Autodesk Inventor part; units mm, degrees
(part 3 of 3)
sketch "Sketch3" plane through (0, 0, 0) normal (-1, 0, 0) x (0, 0, 1)
  line L0 (70.1139, 246.1211) -> (70.1139, 280.6833) projected
  line L1 (70.1139, 280.6833) -> (54.8144, 280.6833) projected
  line L2 (54.8144, 280.6833) -> (54.8144, 296.1211) projected
  line L3 (54.8144, 296.1211) -> (81.2199, 296.1211) projected
  line L4 (81.2199, 296.1211) -> (87.7637, 289.6234) projected
  line L5 (87.7637, 289.6234) -> (87.7637, 252.6188) projected
  line L6 (87.7637, 252.6188) -> (81.266, 246.1211) projected
  line L7 (81.266, 246.1211) -> (70.1139, 246.1211) projected
  line L8 (109.8374, 246.075) -> (109.8374, 261.8815) projected
  line L9 (109.8374, 261.8815) -> (125.1369, 261.8815) projected
  line L10 (125.1369, 261.8815) -> (125.1369, 296.1211) projected
  line L11 (125.1369, 296.1211) -> (142.7867, 296.1211) projected
  line L12 (142.7867, 296.1211) -> (142.7867, 262.6649) projected
  line L13 (142.7867, 262.6649) -> (126.1968, 246.075) projected
  line L14 (126.1968, 246.075) -> (109.8374, 246.075) projected
  line L15 (145.5517, 246.1211) -> (145.5517, 260.9137) projected
  line L16 (145.5517, 260.9137) -> (178.501, 260.9137) projected
  line L17 (178.501, 260.9137) -> (178.501, 246.1211) projected
  line L18 (178.501, 246.1211) -> (145.5517, 246.1211) projected
  line L19 (180.5286, 246.1211) -> (180.5286, 296.1211) projected
  line L20 (180.5286, 296.1211) -> (191.5885, 296.1211) projected
  line L21 (191.5885, 296.1211) -> (198.0862, 289.6234) projected
  line L22 (198.0862, 289.6234) -> (198.0862, 252.6188) projected
  line L23 (198.0862, 252.6188) -> (191.5885, 246.1211) projected
  line L24 (191.5885, 246.1211) -> (180.5286, 246.1211) projected
  line L25 (220.4365, 246.1672) -> (220.4365, 260.9598) projected
  line L26 (220.4365, 260.9598) -> (235.736, 260.9598) projected
  line L27 (235.736, 260.9598) -> (235.736, 282.204) projected
  line L28 (235.736, 282.204) -> (253.3858, 282.204) projected
  line L29 (253.3858, 282.204) -> (253.3858, 254.2317) projected
  line L30 (253.3858, 254.2317) -> (245.3213, 246.1672) projected
  line L31 (245.3213, 246.1672) -> (220.4365, 246.1672) projected
  line L32 (301.9111, 246.1211) -> (290.9895, 246.1211) projected
  line L33 (290.9895, 246.1211) -> (290.9895, 296.1211) projected
  line L34 (290.9895, 296.1211) -> (308.4088, 296.1211) projected
  line L35 (308.4088, 296.1211) -> (308.4088, 252.6188) projected
  line L36 (308.4088, 252.6188) -> (301.9111, 246.1211) projected
  line L37 (288.9618, 246.1211) -> (256.1508, 246.1211) projected
  line L38 (256.1508, 246.1211) -> (256.1508, 260.9137) projected
  line L39 (256.1508, 260.9137) -> (288.9618, 260.9137) projected
  line L40 (288.9618, 260.9137) -> (288.9618, 246.1211) projected
  line L41 (200.8512, 246.1672) -> (200.8512, 282.204) projected
  line L42 (200.8512, 282.204) -> (218.501, 282.204) projected
  line L43 (218.501, 282.204) -> (218.501, 246.1672) projected
  line L44 (218.501, 246.1672) -> (200.8512, 246.1672) projected
  line L45 (145.5517, 280.6833) -> (145.5517, 296.1211) projected
  line L46 (145.5517, 296.1211) -> (178.501, 296.1211) projected
  line L47 (178.501, 296.1211) -> (178.501, 280.6833) projected
  line L48 (178.501, 280.6833) -> (145.5517, 280.6833) projected
  line L49 (145.5517, 266.5358) -> (145.5517, 278.6557) projected
  line L50 (145.5517, 278.6557) -> (178.501, 278.6557) projected
  line L51 (178.501, 278.6557) -> (178.501, 266.5358) projected
  line L52 (178.501, 266.5358) -> (145.5517, 266.5358) projected
  line L53 (107.9019, 246.1211) -> (90.5286, 262.757) projected
  line L54 (90.5286, 262.757) -> (90.5286, 296.1211) projected
  line L55 (90.5286, 296.1211) -> (107.9019, 296.1211) projected
  line L56 (107.9019, 296.1211) -> (107.9019, 246.1211) projected
  line L57 (35.2291, 252.6649) -> (35.2291, 289.5773) projected
  line L58 (35.2291, 289.5773) -> (41.7729, 296.1211) projected
  line L59 (41.7729, 296.1211) -> (52.8789, 296.1211) projected
  line L60 (52.8789, 296.1211) -> (52.8789, 260.9137) projected
  line L61 (52.8789, 260.9137) -> (68.2706, 260.9137) projected
  line L62 (68.2706, 260.9137) -> (68.2706, 246.1211) projected
  line L63 (68.2706, 246.1211) -> (41.7729, 246.1211) projected
  line L64 (41.7729, 246.1211) -> (35.2291, 252.6649) projected
  line L65 (-22.4898, 96.0981) -> (-22.4898, 576.0981) projected
  line L66 (367.5102, 96.0981) -> (-22.4898, 96.0981) projected
  line L67 (367.5102, 576.0981) -> (367.5102, 96.0981) projected
  line L68 (-22.4898, 576.0981) -> (367.5102, 576.0981) projected
  circle A0 centre (42.5102, 103.5981) radius 1.75 projected
  circle A1 centre (302.5102, 568.5981) radius 1.75 projected
  circle A2 centre (42.5102, 568.5981) radius 1.75 projected
  circle A3 centre (360.0102, 161.0981) radius 1.75 projected
  circle A4 centre (360.0102, 511.0981) radius 1.75 projected
  circle A5 centre (-14.9898, 161.0981) radius 1.75 projected
  circle A6 centre (-14.9898, 511.0981) radius 1.75 projected
  circle A7 centre (172.5102, 568.5981) radius 1.75 projected
  circle A8 centre (302.5102, 103.5981) radius 1.75 projected
  line L69 (-2.265, 163.0981) -> (3.5085, 163.0981) projected
  line L70 (-5.1518, 168.0981) -> (-2.265, 163.0981) projected
  line L71 (-2.265, 173.0981) -> (-5.1518, 168.0981) projected
  line L72 (3.5085, 173.0981) -> (-2.265, 173.0981) projected
  line L73 (6.3952, 168.0981) -> (3.5085, 173.0981) projected
  line L74 (3.5085, 163.0981) -> (6.3952, 168.0981) projected
  line L75 (23.735, 143.0981) -> (20.8482, 138.0981) projected
  line L76 (29.5085, 143.0981) -> (23.735, 143.0981) projected
  line L77 (32.3952, 138.0981) -> (29.5085, 143.0981) projected
  line L78 (29.5085, 133.0981) -> (32.3952, 138.0981) projected
  line L79 (23.735, 133.0981) -> (29.5085, 133.0981) projected
  line L80 (20.8482, 138.0981) -> (23.735, 133.0981) projected
  line L81 (45.3856, 160.5981) -> (42.4988, 165.5981) projected
  line L82 (42.4988, 155.5981) -> (45.3856, 160.5981) projected
  line L83 (36.7253, 155.5981) -> (42.4988, 155.5981) projected
  line L84 (33.8386, 160.5981) -> (36.7253, 155.5981) projected
  line L85 (36.7253, 165.5981) -> (33.8386, 160.5981) projected
  line L86 (42.4988, 165.5981) -> (36.7253, 165.5981) projected
  line L87 (55.5085, 128.0981) -> (49.735, 128.0981) projected
  line L88 (58.3952, 123.0981) -> (55.5085, 128.0981) projected
  line L89 (55.5085, 118.0981) -> (58.3952, 123.0981) projected
  line L90 (49.735, 118.0981) -> (55.5085, 118.0981) projected
  line L91 (46.8482, 123.0981) -> (49.735, 118.0981) projected
  line L92 (49.735, 128.0981) -> (46.8482, 123.0981) projected
  line L93 (72.8482, 168.0981) -> (75.735, 163.0981) projected
  line L94 (75.735, 173.0981) -> (72.8482, 168.0981) projected
  line L95 (81.5085, 173.0981) -> (75.735, 173.0981) projected
  line L96 (84.3952, 168.0981) -> (81.5085, 173.0981) projected
  line L97 (81.5085, 163.0981) -> (84.3952, 168.0981) projected
  line L98 (75.735, 163.0981) -> (81.5085, 163.0981) projected
  line L99 (97.3856, 130.5981) -> (94.4988, 135.5981) projected
  line L100 (94.4988, 125.5981) -> (97.3856, 130.5981) projected
  line L101 (88.7253, 125.5981) -> (94.4988, 125.5981) projected
  line L102 (85.8386, 130.5981) -> (88.7253, 125.5981) projected
  line L103 (88.7253, 135.5981) -> (85.8386, 130.5981) projected
  line L104 (94.4988, 135.5981) -> (88.7253, 135.5981) projected
  line L105 (107.5085, 158.0981) -> (101.735, 158.0981) projected
  line L106 (110.3952, 153.0981) -> (107.5085, 158.0981) projected
  line L107 (107.5085, 148.0981) -> (110.3952, 153.0981) projected
  line L108 (101.735, 148.0981) -> (107.5085, 148.0981) projected
  line L109 (98.8482, 153.0981) -> (101.735, 148.0981) projected
  line L110 (101.735, 158.0981) -> (98.8482, 153.0981) projected
  line L111 (120.4988, 140.5981) -> (123.3856, 145.5981) projected
  line L112 (114.7253, 140.5981) -> (120.4988, 140.5981) projected
  line L113 (111.8386, 145.5981) -> (114.7253, 140.5981) projected
  line L114 (114.7253, 150.5981) -> (111.8386, 145.5981) projected
  line L115 (120.4988, 150.5981) -> (114.7253, 150.5981) projected
  line L116 (123.3856, 145.5981) -> (120.4988, 150.5981) projected
  line L117 (127.735, 143.0981) -> (124.8482, 138.0981) projected
  line L118 (133.5085, 143.0981) -> (127.735, 143.0981) projected
  line L119 (136.3952, 138.0981) -> (133.5085, 143.0981) projected
  line L120 (133.5085, 133.0981) -> (136.3952, 138.0981) projected
  line L121 (127.735, 133.0981) -> (133.5085, 133.0981) projected
  line L122 (124.8482, 138.0981) -> (127.735, 133.0981) projected
  line L123 (153.735, 143.0981) -> (150.8482, 138.0981) projected
  line L124 (159.5085, 143.0981) -> (153.735, 143.0981) projected
  line L125 (162.3952, 138.0981) -> (159.5085, 143.0981) projected
  line L126 (159.5085, 133.0981) -> (162.3952, 138.0981) projected
  line L127 (153.735, 133.0981) -> (159.5085, 133.0981) projected
  line L128 (150.8482, 138.0981) -> (153.735, 133.0981) projected
  line L129 (159.5085, 158.0981) -> (153.735, 158.0981) projected
  line L130 (162.3952, 153.0981) -> (159.5085, 158.0981) projected
  line L131 (159.5085, 148.0981) -> (162.3952, 153.0981) projected
  line L132 (153.735, 148.0981) -> (159.5085, 148.0981) projected
  line L133 (150.8482, 153.0981) -> (153.735, 148.0981) projected
  line L134 (153.735, 158.0981) -> (150.8482, 153.0981) projected
  line L135 (176.8482, 168.0981) -> (179.735, 163.0981) projected
  line L136 (179.735, 173.0981) -> (176.8482, 168.0981) projected
  line L137 (185.5085, 173.0981) -> (179.735, 173.0981) projected
  line L138 (188.3952, 168.0981) -> (185.5085, 173.0981) projected
  line L139 (185.5085, 163.0981) -> (188.3952, 168.0981) projected
  line L140 (179.735, 163.0981) -> (185.5085, 163.0981) projected
  line L141 (201.3856, 130.5981) -> (198.4988, 135.5981) projected
  line L142 (198.4988, 125.5981) -> (201.3856, 130.5981) projected
  line L143 (192.7253, 125.5981) -> (198.4988, 125.5981) projected
  line L144 (189.8386, 130.5981) -> (192.7253, 125.5981) projected
  line L145 (192.7253, 135.5981) -> (189.8386, 130.5981) projected
  line L146 (198.4988, 135.5981) -> (192.7253, 135.5981) projected
  line L147 (211.5085, 158.0981) -> (205.735, 158.0981) projected
  line L148 (214.3952, 153.0981) -> (211.5085, 158.0981) projected
  line L149 (211.5085, 148.0981) -> (214.3952, 153.0981) projected
  line L150 (205.735, 148.0981) -> (211.5085, 148.0981) projected
  line L151 (202.8482, 153.0981) -> (205.735, 148.0981) projected
  line L152 (205.735, 158.0981) -> (202.8482, 153.0981) projected
  line L153 (224.4988, 140.5981) -> (227.3856, 145.5981) projected
  line L154 (218.7253, 140.5981) -> (224.4988, 140.5981) projected
  line L155 (215.8386, 145.5981) -> (218.7253, 140.5981) projected
  line L156 (218.7253, 150.5981) -> (215.8386, 145.5981) projected
  line L157 (224.4988, 150.5981) -> (218.7253, 150.5981) projected
  line L158 (227.3856, 145.5981) -> (224.4988, 150.5981) projected
  line L159 (231.735, 143.0981) -> (228.8482, 138.0981) projected
  line L160 (237.5085, 143.0981) -> (231.735, 143.0981) projected
  line L161 (240.3952, 138.0981) -> (237.5085, 143.0981) projected
  line L162 (237.5085, 133.0981) -> (240.3952, 138.0981) projected
  line L163 (231.735, 133.0981) -> (237.5085, 133.0981) projected
  line L164 (228.8482, 138.0981) -> (231.735, 133.0981) projected
  line L165 (253.3856, 160.5981) -> (250.4988, 165.5981) projected
  line L166 (250.4988, 155.5981) -> (253.3856, 160.5981) projected
  line L167 (244.7253, 155.5981) -> (250.4988, 155.5981) projected
  line L168 (241.8386, 160.5981) -> (244.7253, 155.5981) projected
  line L169 (244.7253, 165.5981) -> (241.8386, 160.5981) projected
  line L170 (250.4988, 165.5981) -> (244.7253, 165.5981) projected
  line L171 (263.5085, 128.0981) -> (257.735, 128.0981) projected
  line L172 (266.3952, 123.0981) -> (263.5085, 128.0981) projected
  line L173 (263.5085, 118.0981) -> (266.3952, 123.0981) projected
  line L174 (257.735, 118.0981) -> (263.5085, 118.0981) projected
  line L175 (254.8482, 123.0981) -> (257.735, 118.0981) projected
  line L176 (257.735, 128.0981) -> (254.8482, 123.0981) projected
  line L177 (315.5085, 128.0981) -> (309.735, 128.0981) projected
  line L178 (318.3952, 123.0981) -> (315.5085, 128.0981) projected
  line L179 (315.5085, 118.0981) -> (318.3952, 123.0981) projected
  line L180 (309.735, 118.0981) -> (315.5085, 118.0981) projected
  line L181 (306.8482, 123.0981) -> (309.735, 118.0981) projected
  line L182 (309.735, 128.0981) -> (306.8482, 123.0981) projected
  line L183 (341.5085, 158.0981) -> (335.735, 158.0981) projected
  line L184 (344.3952, 153.0981) -> (341.5085, 158.0981) projected
  line L185 (341.5085, 148.0981) -> (344.3952, 153.0981) projected
  line L186 (335.735, 148.0981) -> (341.5085, 148.0981) projected
  line L187 (332.8482, 153.0981) -> (335.735, 148.0981) projected
  line L188 (335.735, 158.0981) -> (332.8482, 153.0981) projected
  line L189 (280.8482, 168.0981) -> (283.735, 163.0981) projected
  line L190 (283.735, 173.0981) -> (280.8482, 168.0981) projected
  line L191 (289.5085, 173.0981) -> (283.735, 173.0981) projected
  line L192 (292.3952, 168.0981) -> (289.5085, 173.0981) projected
  line L193 (289.5085, 163.0981) -> (292.3952, 168.0981) projected
  line L194 (283.735, 163.0981) -> (289.5085, 163.0981) projected
  line L195 (283.735, 143.0981) -> (280.8482, 138.0981) projected
  line L196 (289.5085, 143.0981) -> (283.735, 143.0981) projected
  line L197 (292.3952, 138.0981) -> (289.5085, 143.0981) projected
  line L198 (289.5085, 133.0981) -> (292.3952, 138.0981) projected
  line L199 (283.735, 133.0981) -> (289.5085, 133.0981) projected
  line L200 (280.8482, 138.0981) -> (283.735, 133.0981) projected
  line L201 (309.735, 143.0981) -> (306.8482, 138.0981) projected
  line L202 (315.5085, 143.0981) -> (309.735, 143.0981) projected
  line L203 (318.3952, 138.0981) -> (315.5085, 143.0981) projected
  line L204 (315.5085, 133.0981) -> (318.3952, 138.0981) projected
  line L205 (309.735, 133.0981) -> (315.5085, 133.0981) projected
  line L206 (306.8482, 138.0981) -> (309.735, 133.0981) projected
  line L207 (3.5085, 128.0981) -> (-2.265, 128.0981) projected
  line L208 (6.3952, 123.0981) -> (3.5085, 128.0981) projected
  line L209 (3.5085, 118.0981) -> (6.3952, 123.0981) projected
  line L210 (-2.265, 118.0981) -> (3.5085, 118.0981) projected
  line L211 (-5.1518, 123.0981) -> (-2.265, 118.0981) projected
  line L212 (-2.265, 128.0981) -> (-5.1518, 123.0981) projected
  line L213 (10.7253, 140.5981) -> (16.4988, 140.5981) projected
  line L214 (7.8386, 145.5981) -> (10.7253, 140.5981) projected
  line L215 (10.7253, 150.5981) -> (7.8386, 145.5981) projected
  line L216 (16.4988, 150.5981) -> (10.7253, 150.5981) projected
  line L217 (19.3856, 145.5981) -> (16.4988, 150.5981) projected
  line L218 (16.4988, 140.5981) -> (19.3856, 145.5981) projected
  line L219 (328.4988, 140.5981) -> (331.3856, 145.5981) projected
  line L220 (322.7253, 140.5981) -> (328.4988, 140.5981) projected
  line L221 (319.8386, 145.5981) -> (322.7253, 140.5981) projected
  line L222 (322.7253, 150.5981) -> (319.8386, 145.5981) projected
  line L223 (328.4988, 150.5981) -> (322.7253, 150.5981) projected
  line L224 (331.3856, 145.5981) -> (328.4988, 150.5981) projected
  line L225 (302.4988, 140.5981) -> (305.3856, 145.5981) projected
  line L226 (296.7253, 140.5981) -> (302.4988, 140.5981) projected
  line L227 (293.8386, 145.5981) -> (296.7253, 140.5981) projected
  line L228 (296.7253, 150.5981) -> (293.8386, 145.5981) projected
  line L229 (302.4988, 150.5981) -> (296.7253, 150.5981) projected
  line L230 (305.3856, 145.5981) -> (302.4988, 150.5981) projected
  line L231 (279.3856, 160.5981) -> (276.4988, 165.5981) projected
  line L232 (276.4988, 155.5981) -> (279.3856, 160.5981) projected
  line L233 (270.7253, 155.5981) -> (276.4988, 155.5981) projected
  line L234 (267.8386, 160.5981) -> (270.7253, 155.5981) projected
  line L235 (270.7253, 165.5981) -> (267.8386, 160.5981) projected
  line L236 (276.4988, 165.5981) -> (270.7253, 165.5981) projected
  line L237 (332.8482, 168.0981) -> (335.735, 163.0981) projected
  line L238 (335.735, 173.0981) -> (332.8482, 168.0981) projected
  line L239 (341.5085, 173.0981) -> (335.735, 173.0981) projected
  line L240 (344.3952, 168.0981) -> (341.5085, 173.0981) projected
  line L241 (341.5085, 163.0981) -> (344.3952, 168.0981) projected
  line L242 (335.735, 163.0981) -> (341.5085, 163.0981) projected
  line L243 (331.3856, 130.5981) -> (328.4988, 135.5981) projected
  line L244 (328.4988, 125.5981) -> (331.3856, 130.5981) projected
  line L245 (322.7253, 125.5981) -> (328.4988, 125.5981) projected
  line L246 (319.8386, 130.5981) -> (322.7253, 125.5981) projected
  line L247 (322.7253, 135.5981) -> (319.8386, 130.5981) projected
  line L248 (328.4988, 135.5981) -> (322.7253, 135.5981) projected
  line L249 (279.3856, 130.5981) -> (276.4988, 135.5981) projected
  line L250 (276.4988, 125.5981) -> (279.3856, 130.5981) projected
  line L251 (270.7253, 125.5981) -> (276.4988, 125.5981) projected
  line L252 (267.8386, 130.5981) -> (270.7253, 125.5981) projected
  line L253 (270.7253, 135.5981) -> (267.8386, 130.5981) projected
  line L254 (276.4988, 135.5981) -> (270.7253, 135.5981) projected
  line L255 (254.8482, 168.0981) -> (257.735, 163.0981) projected
  line L256 (257.735, 173.0981) -> (254.8482, 168.0981) projected
  line L257 (263.5085, 173.0981) -> (257.735, 173.0981) projected
  line L258 (266.3952, 168.0981) -> (263.5085, 173.0981) projected
  line L259 (263.5085, 163.0981) -> (266.3952, 168.0981) projected
  line L260 (257.735, 163.0981) -> (263.5085, 163.0981) projected
  line L261 (237.5085, 128.0981) -> (231.735, 128.0981) projected
  line L262 (240.3952, 123.0981) -> (237.5085, 128.0981) projected
  line L263 (237.5085, 118.0981) -> (240.3952, 123.0981) projected
  line L264 (231.735, 118.0981) -> (237.5085, 118.0981) projected
  line L265 (228.8482, 123.0981) -> (231.735, 118.0981) projected
  line L266 (231.735, 128.0981) -> (228.8482, 123.0981) projected
  line L267 (227.3856, 160.5981) -> (224.4988, 165.5981) projected
  line L268 (224.4988, 155.5981) -> (227.3856, 160.5981) projected
  line L269 (218.7253, 155.5981) -> (224.4988, 155.5981) projected
  line L270 (215.8386, 160.5981) -> (218.7253, 155.5981) projected
  line L271 (218.7253, 165.5981) -> (215.8386, 160.5981) projected
  line L272 (224.4988, 165.5981) -> (218.7253, 165.5981) projected
  line L273 (205.735, 143.0981) -> (202.8482, 138.0981) projected
  line L274 (211.5085, 143.0981) -> (205.735, 143.0981) projected
  line L275 (214.3952, 138.0981) -> (211.5085, 143.0981) projected
  line L276 (211.5085, 133.0981) -> (214.3952, 138.0981) projected
  line L277 (205.735, 133.0981) -> (211.5085, 133.0981) projected
  line L278 (202.8482, 138.0981) -> (205.735, 133.0981) projected
  line L279 (198.4988, 140.5981) -> (201.3856, 145.5981) projected
  line L280 (192.7253, 140.5981) -> (198.4988, 140.5981) projected
  line L281 (189.8386, 145.5981) -> (192.7253, 140.5981) projected
  line L282 (192.7253, 150.5981) -> (189.8386, 145.5981) projected
  line L283 (198.4988, 150.5981) -> (192.7253, 150.5981) projected
  line L284 (201.3856, 145.5981) -> (198.4988, 150.5981) projected
  line L285 (185.5085, 158.0981) -> (179.735, 158.0981) projected
  line L286 (188.3952, 153.0981) -> (185.5085, 158.0981) projected
  line L287 (185.5085, 148.0981) -> (188.3952, 153.0981) projected
  line L288 (179.735, 148.0981) -> (185.5085, 148.0981) projected
  line L289 (176.8482, 153.0981) -> (179.735, 148.0981) projected
  line L290 (179.735, 158.0981) -> (176.8482, 153.0981) projected
  line L291 (175.3856, 130.5981) -> (172.4988, 135.5981) projected
  line L292 (172.4988, 125.5981) -> (175.3856, 130.5981) projected
  line L293 (166.7253, 125.5981) -> (172.4988, 125.5981) projected
  line L294 (163.8386, 130.5981) -> (166.7253, 125.5981) projected
  line L295 (166.7253, 135.5981) -> (163.8386, 130.5981) projected
  line L296 (172.4988, 135.5981) -> (166.7253, 135.5981) projected
  line L297 (146.4988, 140.5981) -> (149.3856, 145.5981) projected
  line L298 (140.7253, 140.5981) -> (146.4988, 140.5981) projected
  line L299 (137.8386, 145.5981) -> (140.7253, 140.5981) projected
  line L300 (140.7253, 150.5981) -> (137.8386, 145.5981) projected
  line L301 (146.4988, 150.5981) -> (140.7253, 150.5981) projected
  line L302 (149.3856, 145.5981) -> (146.4988, 150.5981) projected
  line L303 (133.5085, 128.0981) -> (127.735, 128.0981) projected
  line L304 (136.3952, 123.0981) -> (133.5085, 128.0981) projected
  line L305 (133.5085, 118.0981) -> (136.3952, 123.0981) projected
  line L306 (127.735, 118.0981) -> (133.5085, 118.0981) projected
  line L307 (124.8482, 123.0981) -> (127.735, 118.0981) projected
  line L308 (127.735, 128.0981) -> (124.8482, 123.0981) projected
  line L309 (123.3856, 160.5981) -> (120.4988, 165.5981) projected
  line L310 (120.4988, 155.5981) -> (123.3856, 160.5981) projected
  line L311 (114.7253, 155.5981) -> (120.4988, 155.5981) projected
  line L312 (111.8386, 160.5981) -> (114.7253, 155.5981) projected
  line L313 (114.7253, 165.5981) -> (111.8386, 160.5981) projected
  line L314 (120.4988, 165.5981) -> (114.7253, 165.5981) projected
  line L315 (101.735, 143.0981) -> (98.8482, 138.0981) projected
  line L316 (107.5085, 143.0981) -> (101.735, 143.0981) projected
  line L317 (110.3952, 138.0981) -> (107.5085, 143.0981) projected
  line L318 (107.5085, 133.0981) -> (110.3952, 138.0981) projected
  line L319 (101.735, 133.0981) -> (107.5085, 133.0981) projected
  line L320 (98.8482, 138.0981) -> (101.735, 133.0981) projected
  line L321 (94.4988, 140.5981) -> (97.3856, 145.5981) projected
  line L322 (88.7253, 140.5981) -> (94.4988, 140.5981) projected
  line L323 (85.8386, 145.5981) -> (88.7253, 140.5981) projected
  line L324 (88.7253, 150.5981) -> (85.8386, 145.5981) projected
  line L325 (94.4988, 150.5981) -> (88.7253, 150.5981) projected
  line L326 (97.3856, 145.5981) -> (94.4988, 150.5981) projected
  line L327 (81.5085, 158.0981) -> (75.735, 158.0981) projected
  line L328 (84.3952, 153.0981) -> (81.5085, 158.0981) projected
  line L329 (81.5085, 148.0981) -> (84.3952, 153.0981) projected
  line L330 (75.735, 148.0981) -> (81.5085, 148.0981) projected
  line L331 (72.8482, 153.0981) -> (75.735, 148.0981) projected
  line L332 (75.735, 158.0981) -> (72.8482, 153.0981) projected
  line L333 (71.3856, 130.5981) -> (68.4988, 135.5981) projected
  line L334 (68.4988, 125.5981) -> (71.3856, 130.5981) projected
  line L335 (62.7253, 125.5981) -> (68.4988, 125.5981) projected
  line L336 (59.8386, 130.5981) -> (62.7253, 125.5981) projected
  line L337 (62.7253, 135.5981) -> (59.8386, 130.5981) projected
  line L338 (68.4988, 135.5981) -> (62.7253, 135.5981) projected
  line L339 (46.8482, 168.0981) -> (49.735, 163.0981) projected
  line L340 (49.735, 173.0981) -> (46.8482, 168.0981) projected
  line L341 (55.5085, 173.0981) -> (49.735, 173.0981) projected
  line L342 (58.3952, 168.0981) -> (55.5085, 173.0981) projected
  line L343 (55.5085, 163.0981) -> (58.3952, 168.0981) projected
  line L344 (49.735, 163.0981) -> (55.5085, 163.0981) projected
  line L345 (29.5085, 128.0981) -> (23.735, 128.0981) projected
  line L346 (32.3952, 123.0981) -> (29.5085, 128.0981) projected
  line L347 (29.5085, 118.0981) -> (32.3952, 123.0981) projected
  line L348 (23.735, 118.0981) -> (29.5085, 118.0981) projected
  line L349 (20.8482, 123.0981) -> (23.735, 118.0981) projected
  line L350 (23.735, 128.0981) -> (20.8482, 123.0981) projected
  line L351 (10.7253, 155.5981) -> (16.4988, 155.5981) projected
  line L352 (7.8386, 160.5981) -> (10.7253, 155.5981) projected
  line L353 (10.7253, 165.5981) -> (7.8386, 160.5981) projected
  line L354 (16.4988, 165.5981) -> (10.7253, 165.5981) projected
  line L355 (19.3856, 160.5981) -> (16.4988, 165.5981) projected
  line L356 (16.4988, 155.5981) -> (19.3856, 160.5981) projected
  line L357 (29.5085, 158.0981) -> (23.735, 158.0981) projected
  line L358 (32.3952, 153.0981) -> (29.5085, 158.0981) projected
  line L359 (29.5085, 148.0981) -> (32.3952, 153.0981) projected
  line L360 (23.735, 148.0981) -> (29.5085, 148.0981) projected
  line L361 (20.8482, 153.0981) -> (23.735, 148.0981) projected
  line L362 (23.735, 158.0981) -> (20.8482, 153.0981) projected
  line L363 (42.4988, 140.5981) -> (45.3856, 145.5981) projected
  line L364 (36.7253, 140.5981) -> (42.4988, 140.5981) projected
  line L365 (33.8386, 145.5981) -> (36.7253, 140.5981) projected
  line L366 (36.7253, 150.5981) -> (33.8386, 145.5981) projected
  line L367 (42.4988, 150.5981) -> (36.7253, 150.5981) projected
  line L368 (45.3856, 145.5981) -> (42.4988, 150.5981) projected
  line L369 (49.735, 143.0981) -> (46.8482, 138.0981) projected
  line L370 (55.5085, 143.0981) -> (49.735, 143.0981) projected
  line L371 (58.3952, 138.0981) -> (55.5085, 143.0981) projected
  line L372 (55.5085, 133.0981) -> (58.3952, 138.0981) projected
  line L373 (49.735, 133.0981) -> (55.5085, 133.0981) projected
  line L374 (46.8482, 138.0981) -> (49.735, 133.0981) projected
  line L375 (71.3856, 160.5981) -> (68.4988, 165.5981) projected
  line L376 (68.4988, 155.5981) -> (71.3856, 160.5981) projected
  line L377 (62.7253, 155.5981) -> (68.4988, 155.5981) projected
  line L378 (59.8386, 160.5981) -> (62.7253, 155.5981) projected
  line L379 (62.7253, 165.5981) -> (59.8386, 160.5981) projected
  line L380 (68.4988, 165.5981) -> (62.7253, 165.5981) projected
  line L381 (81.5085, 128.0981) -> (75.735, 128.0981) projected
  line L382 (84.3952, 123.0981) -> (81.5085, 128.0981) projected
  line L383 (81.5085, 118.0981) -> (84.3952, 123.0981) projected
  line L384 (75.735, 118.0981) -> (81.5085, 118.0981) projected
  line L385 (72.8482, 123.0981) -> (75.735, 118.0981) projected
  line L386 (75.735, 128.0981) -> (72.8482, 123.0981) projected
  line L387 (98.8482, 168.0981) -> (101.735, 163.0981) projected
  line L388 (101.735, 173.0981) -> (98.8482, 168.0981) projected
  line L389 (107.5085, 173.0981) -> (101.735, 173.0981) projected
  line L390 (110.3952, 168.0981) -> (107.5085, 173.0981) projected
  line L391 (107.5085, 163.0981) -> (110.3952, 168.0981) projected
  line L392 (101.735, 163.0981) -> (107.5085, 163.0981) projected
  line L393 (123.3856, 130.5981) -> (120.4988, 135.5981) projected
  line L394 (120.4988, 125.5981) -> (123.3856, 130.5981) projected
  line L395 (114.7253, 125.5981) -> (120.4988, 125.5981) projected
  line L396 (111.8386, 130.5981) -> (114.7253, 125.5981) projected
  line L397 (114.7253, 135.5981) -> (111.8386, 130.5981) projected
  line L398 (120.4988, 135.5981) -> (114.7253, 135.5981) projected
  line L399 (133.5085, 158.0981) -> (127.735, 158.0981) projected
  line L400 (136.3952, 153.0981) -> (133.5085, 158.0981) projected
  line L401 (133.5085, 148.0981) -> (136.3952, 153.0981) projected
  line L402 (127.735, 148.0981) -> (133.5085, 148.0981) projected
  line L403 (124.8482, 153.0981) -> (127.735, 148.0981) projected
  line L404 (127.735, 158.0981) -> (124.8482, 153.0981) projected
  line L405 (159.5085, 128.0981) -> (153.735, 128.0981) projected
  line L406 (162.3952, 123.0981) -> (159.5085, 128.0981) projected
  line L407 (159.5085, 118.0981) -> (162.3952, 123.0981) projected
  line L408 (153.735, 118.0981) -> (159.5085, 118.0981) projected
  line L409 (150.8482, 123.0981) -> (153.735, 118.0981) projected
  line L410 (153.735, 128.0981) -> (150.8482, 123.0981) projected
  line L411 (150.8482, 168.0981) -> (153.735, 163.0981) projected
  line L412 (153.735, 173.0981) -> (150.8482, 168.0981) projected
  line L413 (159.5085, 173.0981) -> (153.735, 173.0981) projected
  line L414 (162.3952, 168.0981) -> (159.5085, 173.0981) projected
  line L415 (159.5085, 163.0981) -> (162.3952, 168.0981) projected
  line L416 (153.735, 163.0981) -> (159.5085, 163.0981) projected
  line L417 (175.3856, 160.5981) -> (172.4988, 165.5981) projected
  line L418 (172.4988, 155.5981) -> (175.3856, 160.5981) projected
  line L419 (166.7253, 155.5981) -> (172.4988, 155.5981) projected
  line L420 (163.8386, 160.5981) -> (166.7253, 155.5981) projected
  line L421 (166.7253, 165.5981) -> (163.8386, 160.5981) projected
  line L422 (172.4988, 165.5981) -> (166.7253, 165.5981) projected
  line L423 (185.5085, 128.0981) -> (179.735, 128.0981) projected
  line L424 (188.3952, 123.0981) -> (185.5085, 128.0981) projected
  line L425 (185.5085, 118.0981) -> (188.3952, 123.0981) projected
  line L426 (179.735, 118.0981) -> (185.5085, 118.0981) projected
  line L427 (176.8482, 123.0981) -> (179.735, 118.0981) projected
  line L428 (179.735, 128.0981) -> (176.8482, 123.0981) projected
  line L429 (202.8482, 168.0981) -> (205.735, 163.0981) projected
  line L430 (205.735, 173.0981) -> (202.8482, 168.0981) projected
  line L431 (211.5085, 173.0981) -> (205.735, 173.0981) projected
  line L432 (214.3952, 168.0981) -> (211.5085, 173.0981) projected
  line L433 (211.5085, 163.0981) -> (214.3952, 168.0981) projected
  line L434 (205.735, 163.0981) -> (211.5085, 163.0981) projected
  line L435 (227.3856, 130.5981) -> (224.4988, 135.5981) projected
  line L436 (224.4988, 125.5981) -> (227.3856, 130.5981) projected
  line L437 (218.7253, 125.5981) -> (224.4988, 125.5981) projected
  line L438 (215.8386, 130.5981) -> (218.7253, 125.5981) projected
  line L439 (218.7253, 135.5981) -> (215.8386, 130.5981) projected
  line L440 (224.4988, 135.5981) -> (218.7253, 135.5981) projected
  line L441 (237.5085, 158.0981) -> (231.735, 158.0981) projected
  line L442 (240.3952, 153.0981) -> (237.5085, 158.0981) projected
  line L443 (237.5085, 148.0981) -> (240.3952, 153.0981) projected
  line L444 (231.735, 148.0981) -> (237.5085, 148.0981) projected
  line L445 (228.8482, 153.0981) -> (231.735, 148.0981) projected
  line L446 (231.735, 158.0981) -> (228.8482, 153.0981) projected
  line L447 (250.4988, 140.5981) -> (253.3856, 145.5981) projected
  line L448 (244.7253, 140.5981) -> (250.4988, 140.5981) projected
  line L449 (241.8386, 145.5981) -> (244.7253, 140.5981) projected
  line L450 (244.7253, 150.5981) -> (241.8386, 145.5981) projected
  line L451 (250.4988, 150.5981) -> (244.7253, 150.5981) projected
  line L452 (253.3856, 145.5981) -> (250.4988, 150.5981) projected
  line L453 (257.735, 143.0981) -> (254.8482, 138.0981) projected
  line L454 (263.5085, 143.0981) -> (257.735, 143.0981) projected
  line L455 (266.3952, 138.0981) -> (263.5085, 143.0981) projected
  line L456 (263.5085, 133.0981) -> (266.3952, 138.0981) projected
  line L457 (257.735, 133.0981) -> (263.5085, 133.0981) projected
  line L458 (254.8482, 138.0981) -> (257.735, 133.0981) projected
  line L459 (305.3856, 130.5981) -> (302.4988, 135.5981) projected
  line L460 (302.4988, 125.5981) -> (305.3856, 130.5981) projected
  line L461 (296.7253, 125.5981) -> (302.4988, 125.5981) projected
  line L462 (293.8386, 130.5981) -> (296.7253, 125.5981) projected
  line L463 (296.7253, 135.5981) -> (293.8386, 130.5981) projected
  line L464 (302.4988, 135.5981) -> (296.7253, 135.5981) projected
  line L465 (335.735, 143.0981) -> (332.8482, 138.0981) projected
  line L466 (341.5085, 143.0981) -> (335.735, 143.0981) projected
  line L467 (344.3952, 138.0981) -> (341.5085, 143.0981) projected
  line L468 (341.5085, 133.0981) -> (344.3952, 138.0981) projected
  line L469 (335.735, 133.0981) -> (341.5085, 133.0981) projected
  line L470 (332.8482, 138.0981) -> (335.735, 133.0981) projected
  line L471 (306.8482, 168.0981) -> (309.735, 163.0981) projected
  line L472 (309.735, 173.0981) -> (306.8482, 168.0981) projected
  line L473 (315.5085, 173.0981) -> (309.735, 173.0981) projected
  line L474 (318.3952, 168.0981) -> (315.5085, 173.0981) projected
  line L475 (315.5085, 163.0981) -> (318.3952, 168.0981) projected
  line L476 (309.735, 163.0981) -> (315.5085, 163.0981) projected
  line L477 (289.5085, 158.0981) -> (283.735, 158.0981) projected
  line L478 (292.3952, 153.0981) -> (289.5085, 158.0981) projected
  line L479 (289.5085, 148.0981) -> (292.3952, 153.0981) projected
  line L480 (283.735, 148.0981) -> (289.5085, 148.0981) projected
  line L481 (280.8482, 153.0981) -> (283.735, 148.0981) projected
  line L482 (283.735, 158.0981) -> (280.8482, 153.0981) projected
  line L483 (315.5085, 158.0981) -> (309.735, 158.0981) projected
  line L484 (318.3952, 153.0981) -> (315.5085, 158.0981) projected
  line L485 (315.5085, 148.0981) -> (318.3952, 153.0981) projected
  line L486 (309.735, 148.0981) -> (315.5085, 148.0981) projected
  line L487 (306.8482, 153.0981) -> (309.735, 148.0981) projected
  line L488 (309.735, 158.0981) -> (306.8482, 153.0981) projected
  line L489 (-2.265, 148.0981) -> (3.5085, 148.0981) projected
  line L490 (-5.1518, 153.0981) -> (-2.265, 148.0981) projected
  line L491 (-2.265, 158.0981) -> (-5.1518, 153.0981) projected
  line L492 (3.5085, 158.0981) -> (-2.265, 158.0981) projected
  line L493 (6.3952, 153.0981) -> (3.5085, 158.0981) projected
  line L494 (3.5085, 148.0981) -> (6.3952, 153.0981) projected
  line L495 (19.3856, 130.5981) -> (16.4988, 135.5981) projected
  line L496 (16.4988, 125.5981) -> (19.3856, 130.5981) projected
  line L497 (10.7253, 125.5981) -> (16.4988, 125.5981) projected
  line L498 (7.8386, 130.5981) -> (10.7253, 125.5981) projected
  line L499 (10.7253, 135.5981) -> (7.8386, 130.5981) projected
  line L500 (16.4988, 135.5981) -> (10.7253, 135.5981) projected
  line L501 (3.5085, 143.0981) -> (-2.265, 143.0981) projected
  line L502 (6.3952, 138.0981) -> (3.5085, 143.0981) projected
  line L503 (3.5085, 133.0981) -> (6.3952, 138.0981) projected
  line L504 (-2.265, 133.0981) -> (3.5085, 133.0981) projected
  line L505 (-5.1518, 138.0981) -> (-2.265, 133.0981) projected
  line L506 (-2.265, 143.0981) -> (-5.1518, 138.0981) projected
  line L507 (305.3856, 160.5981) -> (302.4988, 165.5981) projected
  line L508 (302.4988, 155.5981) -> (305.3856, 160.5981) projected
  line L509 (296.7253, 155.5981) -> (302.4988, 155.5981) projected
  line L510 (293.8386, 160.5981) -> (296.7253, 155.5981) projected
  line L511 (296.7253, 165.5981) -> (293.8386, 160.5981) projected
  line L512 (302.4988, 165.5981) -> (296.7253, 165.5981) projected
  line L513 (276.4988, 140.5981) -> (279.3856, 145.5981) projected
  line L514 (270.7253, 140.5981) -> (276.4988, 140.5981) projected
  line L515 (267.8386, 145.5981) -> (270.7253, 140.5981) projected
  line L516 (270.7253, 150.5981) -> (267.8386, 145.5981) projected
  line L517 (276.4988, 150.5981) -> (270.7253, 150.5981) projected
  line L518 (279.3856, 145.5981) -> (276.4988, 150.5981) projected
  line L519 (331.3856, 160.5981) -> (328.4988, 165.5981) projected
  line L520 (328.4988, 155.5981) -> (331.3856, 160.5981) projected
  line L521 (322.7253, 155.5981) -> (328.4988, 155.5981) projected
  line L522 (319.8386, 160.5981) -> (322.7253, 155.5981) projected
  line L523 (322.7253, 165.5981) -> (319.8386, 160.5981) projected
  line L524 (328.4988, 165.5981) -> (322.7253, 165.5981) projected
  line L525 (341.5085, 128.0981) -> (335.735, 128.0981) projected
  line L526 (344.3952, 123.0981) -> (341.5085, 128.0981) projected
  line L527 (341.5085, 118.0981) -> (344.3952, 123.0981) projected
  line L528 (335.735, 118.0981) -> (341.5085, 118.0981) projected
  line L529 (332.8482, 123.0981) -> (335.735, 118.0981) projected
  line L530 (335.735, 128.0981) -> (332.8482, 123.0981) projected
  line L531 (289.5085, 128.0981) -> (283.735, 128.0981) projected
  line L532 (292.3952, 123.0981) -> (289.5085, 128.0981) projected
  line L533 (289.5085, 118.0981) -> (292.3952, 123.0981) projected
  line L534 (283.735, 118.0981) -> (289.5085, 118.0981) projected
  line L535 (280.8482, 123.0981) -> (283.735, 118.0981) projected
  line L536 (283.735, 128.0981) -> (280.8482, 123.0981) projected
  line L537 (263.5085, 158.0981) -> (257.735, 158.0981) projected
  line L538 (266.3952, 153.0981) -> (263.5085, 158.0981) projected
  line L539 (263.5085, 148.0981) -> (266.3952, 153.0981) projected
  line L540 (257.735, 148.0981) -> (263.5085, 148.0981) projected
  line L541 (254.8482, 153.0981) -> (257.735, 148.0981) projected
  line L542 (257.735, 158.0981) -> (254.8482, 153.0981) projected
  line L543 (253.3856, 130.5981) -> (250.4988, 135.5981) projected
  line L544 (250.4988, 125.5981) -> (253.3856, 130.5981) projected
  line L545 (244.7253, 125.5981) -> (250.4988, 125.5981) projected
  line L546 (241.8386, 130.5981) -> (244.7253, 125.5981) projected
  line L547 (244.7253, 135.5981) -> (241.8386, 130.5981) projected
  line L548 (250.4988, 135.5981) -> (244.7253, 135.5981) projected
  line L549 (228.8482, 168.0981) -> (231.735, 163.0981) projected
  line L550 (231.735, 173.0981) -> (228.8482, 168.0981) projected
  line L551 (237.5085, 173.0981) -> (231.735, 173.0981) projected
  line L552 (240.3952, 168.0981) -> (237.5085, 173.0981) projected
  line L553 (237.5085, 163.0981) -> (240.3952, 168.0981) projected
  line L554 (231.735, 163.0981) -> (237.5085, 163.0981) projected
  line L555 (211.5085, 128.0981) -> (205.735, 128.0981) projected
  line L556 (214.3952, 123.0981) -> (211.5085, 128.0981) projected
  line L557 (211.5085, 118.0981) -> (214.3952, 123.0981) projected
  line L558 (205.735, 118.0981) -> (211.5085, 118.0981) projected
  line L559 (202.8482, 123.0981) -> (205.735, 118.0981) projected
  line L560 (205.735, 128.0981) -> (202.8482, 123.0981) projected
  line L561 (201.3856, 160.5981) -> (198.4988, 165.5981) projected
  line L562 (198.4988, 155.5981) -> (201.3856, 160.5981) projected
  line L563 (192.7253, 155.5981) -> (198.4988, 155.5981) projected
  line L564 (189.8386, 160.5981) -> (192.7253, 155.5981) projected
  line L565 (192.7253, 165.5981) -> (189.8386, 160.5981) projected
  line L566 (198.4988, 165.5981) -> (192.7253, 165.5981) projected
  line L567 (179.735, 143.0981) -> (176.8482, 138.0981) projected
  line L568 (185.5085, 143.0981) -> (179.735, 143.0981) projected
  line L569 (188.3952, 138.0981) -> (185.5085, 143.0981) projected
  line L570 (185.5085, 133.0981) -> (188.3952, 138.0981) projected
  line L571 (179.735, 133.0981) -> (185.5085, 133.0981) projected
  line L572 (176.8482, 138.0981) -> (179.735, 133.0981) projected
  line L573 (172.4988, 140.5981) -> (175.3856, 145.5981) projected
  line L574 (166.7253, 140.5981) -> (172.4988, 140.5981) projected
  line L575 (163.8386, 145.5981) -> (166.7253, 140.5981) projected
  line L576 (166.7253, 150.5981) -> (163.8386, 145.5981) projected
  line L577 (172.4988, 150.5981) -> (166.7253, 150.5981) projected
  line L578 (175.3856, 145.5981) -> (172.4988, 150.5981) projected
  line L579 (149.3856, 160.5981) -> (146.4988, 165.5981) projected
  line L580 (146.4988, 155.5981) -> (149.3856, 160.5981) projected
  line L581 (140.7253, 155.5981) -> (146.4988, 155.5981) projected
  line L582 (137.8386, 160.5981) -> (140.7253, 155.5981) projected
  line L583 (140.7253, 165.5981) -> (137.8386, 160.5981) projected
  line L584 (146.4988, 165.5981) -> (140.7253, 165.5981) projected
  line L585 (149.3856, 130.5981) -> (146.4988, 135.5981) projected
  line L586 (146.4988, 125.5981) -> (149.3856, 130.5981) projected
  line L587 (140.7253, 125.5981) -> (146.4988, 125.5981) projected
  line L588 (137.8386, 130.5981) -> (140.7253, 125.5981) projected
  line L589 (140.7253, 135.5981) -> (137.8386, 130.5981) projected
  line L590 (146.4988, 135.5981) -> (140.7253, 135.5981) projected
  line L591 (124.8482, 168.0981) -> (127.735, 163.0981) projected
  line L592 (127.735, 173.0981) -> (124.8482, 168.0981) projected
  line L593 (133.5085, 173.0981) -> (127.735, 173.0981) projected
  line L594 (136.3952, 168.0981) -> (133.5085, 173.0981) projected
  line L595 (133.5085, 163.0981) -> (136.3952, 168.0981) projected
  line L596 (127.735, 163.0981) -> (133.5085, 163.0981) projected
  line L597 (107.5085, 128.0981) -> (101.735, 128.0981) projected
  line L598 (110.3952, 123.0981) -> (107.5085, 128.0981) projected
  line L599 (107.5085, 118.0981) -> (110.3952, 123.0981) projected
  line L600 (101.735, 118.0981) -> (107.5085, 118.0981) projected
  line L601 (98.8482, 123.0981) -> (101.735, 118.0981) projected
  line L602 (101.735, 128.0981) -> (98.8482, 123.0981) projected
  line L603 (97.3856, 160.5981) -> (94.4988, 165.5981) projected
  line L604 (94.4988, 155.5981) -> (97.3856, 160.5981) projected
  line L605 (88.7253, 155.5981) -> (94.4988, 155.5981) projected
  line L606 (85.8386, 160.5981) -> (88.7253, 155.5981) projected
  line L607 (88.7253, 165.5981) -> (85.8386, 160.5981) projected
  line L608 (94.4988, 165.5981) -> (88.7253, 165.5981) projected
  line L609 (75.735, 143.0981) -> (72.8482, 138.0981) projected
  line L610 (81.5085, 143.0981) -> (75.735, 143.0981) projected
  line L611 (84.3952, 138.0981) -> (81.5085, 143.0981) projected
  line L612 (81.5085, 133.0981) -> (84.3952, 138.0981) projected
  line L613 (75.735, 133.0981) -> (81.5085, 133.0981) projected
  line L614 (72.8482, 138.0981) -> (75.735, 133.0981) projected
  line L615 (68.4988, 140.5981) -> (71.3856, 145.5981) projected
  line L616 (62.7253, 140.5981) -> (68.4988, 140.5981) projected
  line L617 (59.8386, 145.5981) -> (62.7253, 140.5981) projected
  line L618 (62.7253, 150.5981) -> (59.8386, 145.5981) projected
  line L619 (68.4988, 150.5981) -> (62.7253, 150.5981) projected
  line L620 (71.3856, 145.5981) -> (68.4988, 150.5981) projected
  line L621 (55.5085, 158.0981) -> (49.735, 158.0981) projected
  line L622 (58.3952, 153.0981) -> (55.5085, 158.0981) projected
  line L623 (55.5085, 148.0981) -> (58.3952, 153.0981) projected
  line L624 (49.735, 148.0981) -> (55.5085, 148.0981) projected
  line L625 (46.8482, 153.0981) -> (49.735, 148.0981) projected
  line L626 (49.735, 158.0981) -> (46.8482, 153.0981) projected
  line L627 (45.3856, 130.5981) -> (42.4988, 135.5981) projected
  line L628 (42.4988, 125.5981) -> (45.3856, 130.5981) projected
  line L629 (36.7253, 125.5981) -> (42.4988, 125.5981) projected
  line L630 (33.8386, 130.5981) -> (36.7253, 125.5981) projected
  line L631 (36.7253, 135.5981) -> (33.8386, 130.5981) projected
  line L632 (42.4988, 135.5981) -> (36.7253, 135.5981) projected
  line L633 (20.8482, 168.0981) -> (23.735, 163.0981) projected
  line L634 (23.735, 173.0981) -> (20.8482, 168.0981) projected
  line L635 (29.5085, 173.0981) -> (23.735, 173.0981) projected
  line L636 (32.3952, 168.0981) -> (29.5085, 173.0981) projected
  line L637 (29.5085, 163.0981) -> (32.3952, 168.0981) projected
  line L638 (23.735, 163.0981) -> (29.5085, 163.0981) projected
  line L639 (-7.4898, 496.0981) -> (-13.4898, 496.0981) projected
  point P0 (0, 0)
  point P1 (152.5102, 376.0981)
  point P2 (177.5102, 376.0981)
  point P3 (177.5102, 351.0981)
  point P4 (152.5102, 351.0981)
  point P5 (-10.4898, 496.0981)
  point P6 (147.5102, 526.0981)
  point P7 (197.5102, 526.0981)
  dimension "d6" = 120
  dimension "d7" = 25
  dimension "d8" = 25
  dimension "d9" = 175
  dimension "d17" = 25
  dimension "d18" = 25
  dimension "d19" = 50
  constraints: 3 horizontal alignment, 2 vertical alignment, 1 midpoint
  measures "d6" vertical distance of point (-10.49, 496.098) point (152.51, 376.098)
  measures "d7" distance of point (152.51, 351.098) point (152.51, 376.098)
  measures "d8" distance of point (177.51, 376.098) point (152.51, 376.098)
  measures "d9" distance from line of L65 point (152.51, 376.098)
  measures "d17" horizontal distance of point (147.51, 526.098) A7.centre
  measures "d18" horizontal distance of A7.centre point (197.51, 526.098)
  measures "d19" distance from line of L68 point (147.51, 526.098)
hole "Hole1" at (0, 376.0981, 152.5102) at (0, 376.0981, 177.5102) at (0, 351.0981, 177.5102) at (0, 351.0981, 152.5102) at (0, 526.0981, 197.5102) at (0, 526.0981, 147.5102) direction (1, 0, 0) diameter 3.2 end through all
body "Solid1"
